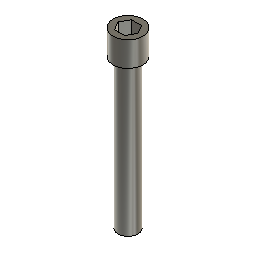
FINAL (Autodesk Fusion 360 archive; units mm, degrees)
design "screw beam"
Autodesk Fusion 360 part; units mm, degrees
sketch "Sketch1" plane through (0, 0, 0) normal (0, 1, 0) x (1, 0, 0)
  line L0 (0, -60) -> (3, -60)
  line L1 (3, -60) -> (3, -55)
  line L2 (3, -55) -> (2, -55)
  line L3 (2, -55) -> (2, -25)
  line L4 (0, -60) -> (0, -25)
  line L5 (0, -25) -> (2, -25)
  dimension "d1" = 3
  dimension "d2" = 5
  dimension "d3" = 1
  dimension "d4" = 30
  dimension "d5" = 35
  constraint horizontal L0
  constraint perpendicular L0 L1
  constraint perpendicular L1 L2
  constraint perpendicular L2 L3
  constraint perpendicular L0 L4
  measures "d1" distance of L0.start L0.end
  measures "d2" distance of L0.end L1.end
  measures "d3" distance of L1.end L2.end
  measures "d4" distance of L2.end L3.end
  measures "d5" distance of L0.start L4.end
revolve "Revolve1" add sketch "Sketch1" angle 360 about axis through (0, 0, 60) along (0, 0, -1)
sketch "Sketch2" plane through (0, 0, 60) normal (0, 0, 1) x (-1, 0, 0)
  circle A0 centre (0, 0) radius 3
  line L0 (1.0047, -1.7293) -> (2, 0.0055)
  line L1 (2, 0.0055) -> (0.9953, 1.7348)
  line L2 (0.9953, 1.7348) -> (-1.0047, 1.7293)
  line L3 (-1.0047, 1.7293) -> (-2, -0.0055)
  line L4 (-2, -0.0055) -> (-0.9953, -1.7348)
  line L5 (-0.9953, -1.7348) -> (1.0047, -1.7293)
  dimension "d7" = 2
  constraint coincident A0.centre origin
  measures "d7" distance of L0.start A0.centre
extrude "Extrude1" cut sketch "Sketch2" against normal blind 5 contours L0 L1 L2 L3 L4 L5

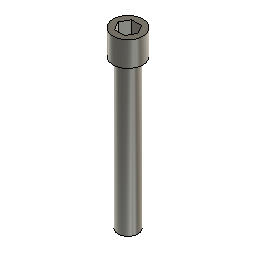
design "screw beam"
Autodesk Fusion 360 part; units mm, degrees
sketch "Sketch1" plane through (0, 0, 0) normal (0, 1, 0) x (1, 0, 0)
  line L0 (0, -60) -> (3, -60)
  line L1 (3, -60) -> (3, -55)
  line L2 (3, -55) -> (2, -55)
  line L3 (2, -55) -> (2, -25)
  line L4 (0, -60) -> (0, -25)
  line L5 (0, -25) -> (2, -25)
  dimension "d1" = 3
  dimension "d2" = 5
  dimension "d3" = 1
  dimension "d4" = 30
  dimension "d5" = 35
  constraint horizontal L0
  constraint perpendicular L0 L1
  constraint perpendicular L1 L2
  constraint perpendicular L2 L3
  constraint perpendicular L0 L4
  measures "d1" distance of L0.start L0.end
  measures "d2" distance of L0.end L1.end
  measures "d3" distance of L1.end L2.end
  measures "d4" distance of L2.end L3.end
  measures "d5" distance of L0.start L4.end
revolve "Revolve1" add sketch "Sketch1" angle 360 about axis through (0, 0, 60) along (0, 0, -1)
sketch "Sketch2" plane through (0, 0, 60) normal (0, 0, 1) x (-1, 0, 0)
  circle A0 centre (0, 0) radius 3
  line L0 (1.0047, -1.7293) -> (2, 0.0055)
  line L1 (2, 0.0055) -> (0.9953, 1.7348)
  line L2 (0.9953, 1.7348) -> (-1.0047, 1.7293)
  line L3 (-1.0047, 1.7293) -> (-2, -0.0055)
  line L4 (-2, -0.0055) -> (-0.9953, -1.7348)
  line L5 (-0.9953, -1.7348) -> (1.0047, -1.7293)
  dimension "d7" = 2
  constraint coincident A0.centre origin
  measures "d7" distance of L0.start A0.centre
extrude "Extrude1" cut sketch "Sketch2" against normal blind 5 contours L0 L1 L2 L3 L4 L5

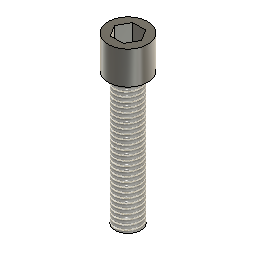
design "Untitled"
Autodesk Fusion 360 part; units mm, degrees
sketch "Sketch1" plane through (0, 0, 0) normal (0, 1, 0) x (1, 0, 0)
sketch "Sketch2" plane through (0, 0, 0) normal (0, 1, 0) x (1, 0, 0)
sketch "Sketch3" plane through (0, 0, 0) normal (0, 1, 0) x (1, 0, 0)
sketch "Sketch4" plane through (0, 0, 0) normal (0, 1, 0) x (1, 0, 0)
sketch "Sketch5" plane through (0, 0, 0) normal (0, 1, 0) x (1, 0, 0)
sketch "Sketch6" plane through (0, 0, 0) normal (0, 1, 0) x (1, 0, 0)
sketch "Sketch7" plane through (0, 0, 0) normal (0, 1, 0) x (1, 0, 0)
sketch "Sketch8" plane through (0, 0, 0) normal (0, 1, 0) x (1, 0, 0)
  line L0 (0, -125) -> (3, -125)
  line L1 (3, -125) -> (3, -120)
  line L2 (3, -120) -> (2, -120)
  line L3 (2, -120) -> (2, -100)
  line L4 (2, -100) -> (0, -100)
  line L5 (0, -100) -> (0, -125)
  dimension "d5" = 3
  dimension "d6" = 5
  dimension "d7" = 1
  dimension "d8" = 20
  constraint horizontal L0
  constraint perpendicular L0 L1
  constraint perpendicular L1 L2
  constraint perpendicular L2 L3
  constraint perpendicular L3 L4
  constraint perpendicular L0 L5
  measures "d5" distance of L0.start L0.end
  measures "d6" distance of L0.end L1.end
  measures "d7" distance of L1.end L2.end
  measures "d8" distance of L2.end L3.end
revolve "Revolve1" add sketch "Sketch8" angle 360 about axis through (0, 0, 100) along (0, 0, 1)
sketch "Sketch9" plane through (0, 0, 125) normal (0, 0, 1) x (-1, 0, 0)
  circle A0 centre (0, 0) radius 3
  line L0 (-1.0132, 1.7244) -> (-1.9999, -0.0153)
  line L1 (-1.9999, -0.0153) -> (-0.9868, -1.7396)
  line L2 (-0.9868, -1.7396) -> (1.0132, -1.7244)
  line L3 (1.0132, -1.7244) -> (1.9999, 0.0153)
  line L4 (1.9999, 0.0153) -> (0.9868, 1.7396)
  line L5 (0.9868, 1.7396) -> (-1.0132, 1.7244)
  dimension "d10" = 2
  constraint coincident A0.centre origin
  measures "d10" distance of L0.start A0.centre
thread "Thread1" "ISO Metric profile 4.0 M4x0.7 6g" major diameter 3.908 minor diameter 3.111 pitch 0.7 angle 60 resizes the face on face at (1.9975, -0.0997, 113.3333)
extrude "Extrude1" cut sketch "Sketch9" against normal blind 5 contours L0 L1 L2 L3 L4 L5
